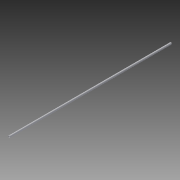
# Autodesk Inventor part: pvcSection
Saved by Autodesk Inventor 2014 (Build 180170000, 170)
## iProperties
Created: 2015-03-27
Part Number: pvcSection
Material: PVC-Piping
Document SubType Name: Modeling
Designer: ddeboer
Mass: 2958.21 g
Surface Area: 10817.7 cm^2
Volume: 2113.01 cm^3
Density: 1.4 g/cm^3
Appearance: Smooth - White
Author: ddeboer
Autodesk Inventor part; units mm, degrees
ref_plane "YZ Plane" through (0, 0, 0) normal (1, 0, 0) x (0, 1, 0)
ref_plane "XZ Plane" through (0, 0, 0) normal (0, 1, 0) x (-1, 0, 0)
ref_plane "XY Plane" through (0, 0, 0) normal (0, 0, 1) x (1, 0, 0)
sketch "Sketch1" plane through (0, 0, 0) normal (0, 0, 1) x (1, 0, 0)
  circle A0 centre (0, 0) radius 31.5
  circle A1 centre (0, 0) radius 28.5
  dimension "d0" = 63
  dimension "d1" = 3
  constraints: 2 centre point, 1 coincident
  measures "d0" diameter of A0
  measures "d1" radial gap between concentric circles of A1 A0
extrude "Extrusion1" add sketch "Sketch1" along normal blind 6000
sketch "Sketch2" plane through (0, 0, 6000) normal (0, 0, 1) x (1, 0, 0)
  circle A0 centre (0, 0) radius 28.5 projected
  circle A1 centre (0, 0) radius 31.5 projected
extrude "Extrusion2" cut sketch "Sketch2" against normal blind 500
sketch "Sketch3" plane through (0, 0, 0) normal (0, 1, 0) x (-1, 0, 0)
  circle A0 centre (0, 2140) radius 0.5
  point P0 (0, 0)
  dimension "d6" = 1
  constraints: 1 centre point
  measures "d6" diameter of A0
hole "overlap2" at (0, 0, 2140) direction (0, -1, 0) diameter 1 end through all
sketch "Sketch4" plane through (0, 0, 0) normal (0, 1, 0) x (-1, 0, 0)
  circle A0 centre (0, 3260) radius 0.5
  point P0 (0, 0)
  dimension "d14" = 1
  constraints: 1 centre point
  measures "d14" diameter of A0
hole "overlap3" at (0, 0, 3260) direction (0, -1, 0) diameter 1 end through all
sketch "Sketch5" plane through (0, 0, 0) normal (0, 1, 0) x (-1, 0, 0)
  circle A0 centre (0, 4400) radius 0.5
  point P0 (0, 0)
  dimension "d22" = 1
  constraints: 1 centre point
  measures "d22" diameter of A0
hole "overlap4" at (0, 0, 4400) direction (0, -1, 0) diameter 1 end through all
sketch "Sketch6" plane through (0, 0, 0) normal (0, 1, 0) x (-1, 0, 0)
  circle A0 centre (0, 5330) radius 3.5
  point P0 (0, 0)
  dimension "d30" = 7
  constraints: 1 centre point
  measures "d30" diameter of A0
extrude "endHole" cut sketch "Sketch6" along normal mid plane 100
sketch "Sketch7" plane through (0, 0, 0) normal (0, 1, 0) x (-1, 0, 0)
  circle A0 centre (0, 100) radius 0.5
  point P0 (0, 0)
  dimension "d33" = 1
  constraints: 1 centre point
  measures "d33" diameter of A0
hole "Hole4" at (0, 0, 100) direction (0, 1, 0) diameter 1 end through all
pattern_linear "Rectangular Pattern1" count 18 spacing 300 along (0, 0, 1) of "Hole4"
body "Solid1"
